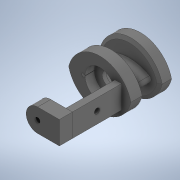
# Autodesk Inventor part: SpoolHolder
Saved by Autodesk Inventor 2022 (Build 260153000, 153)
## iProperties
Created: 2020-03-10
Part Number: SpoolHolder
Material: Generic
Document SubType Name: Modeling
Designer: elmar
Density: 1 g/cm^3
Appearance: Gray
GuideRadius: 25.000 mm
SpoolHolderPlateDiameter: 30.000 mm
CarriageGuideWidth: 10.000 mm
Author: elmar
Autodesk Inventor part; units mm, degrees
ref_plane "YZ Plane" through (0, 0, 0) normal (1, 0, 0) x (0, 1, 0)
ref_plane "XZ Plane" through (0, 0, 0) normal (0, 1, 0) x (-1, 0, 0)
ref_plane "XY Plane" through (0, 0, 0) normal (0, 0, 1) x (1, 0, 0)
sketch "Sketch1" plane through (0, 0, 0) normal (0, 0, 1) x (1, 0, 0)
  circle A0 centre (0, 0) radius 15
  arc A1 (19, 0) -> (-19, 0) centre (0, -4.5333) ccw
  arc A2 (-19, 0) -> (19, 0) centre (0, 4.5333) ccw
  line L0 (-26.6, 0) -> (26.6, 0) projected
  line L1 (0, -21) -> (0, 21) projected
  point P0 (0, 15)
  point P1 (0, -15)
  dimension "SpoolHolderPlateDiameter" = 30
  dimension "d253" = 38
  constraints: 4 point on circle, 3 centre point, 3 point on line, 2 tangent, 1 coincident
  measures "SpoolHolderPlateDiameter" diameter of A0
  measures "d253" distance of A1.end A1.start
extrude "Extrusion1" add sketch "Sketch1" against normal blind 8
sketch "Sketch3" plane through (0, 0, 0) normal (0, 0, -1) x (-1, 0, 0)
  line L0 (-13.2665, 7) -> (-9.2665, 7)
  line L1 (-9.2665, 7) -> (-9.2665, -7)
  line L2 (-9.2665, -7) -> (-13.2665, -7)
  line L3 (-13.2665, -7) -> (-13.2665, 7)
  line L4 (26.6, 0) -> (-26.6, 0) projected
  arc A0 (19, 0) -> (-19, 0) centre (0, -4.5333) ccw projected
  circle A1 centre (0, 0) radius 15
  point P0 (-13.2665, 0)
  dimension "SupportThickness" = 4
  dimension "d254" = 14
  constraints: 8 end point, 2 parallel, 1 coincident, 1 horizontal, 1 midpoint, 1 perpendicular, 1 point on line, 4 other
  measures "SupportThickness" distance of L0.start L0.end
  measures "d254" distance of L0.end L1.end
extrude "Extrusion2" add sketch "Sketch3" against normal blind 30 contours L0 L1 L4 L3 | L4 L1 L2 L3
sketch "Sketch4" plane through (13.2665, 0, -8) normal (1, 0, 0) x (0, 0, 1)
  line L0 (38, 7) -> (38, -7) projected
  line L1 (38, 0) -> (23, 0)
  point P0 (8, 0)
  dimension "HoleHeight" = 15
  constraints: 2 end point, 1 horizontal, 1 midpoint
  measures "HoleHeight" distance of L1.start L1.end
hole "Hole2" at (13.2665, 0, 15) direction (-1, 0, 0) diameter 3.2 depth 4 tip angle 118 clearance for "Flat Head Machine Screw" size "M3" standard "Ansi Metric M Profile"
sketch "Sketch5" plane through (-9.2769, -6.9803, 30) normal (0, 0, 1) x (-1, 0, 0)
  line L0 (-22.5434, -13.9803) -> (-18.5434, -13.9803) projected
  line L1 (-22.5434, 0.0197) -> (-22.5434, -13.9803) projected
  line L2 (-18.5434, 0.0197) -> (-22.5434, 0.0197) projected
  line L3 (-18.5434, -13.9803) -> (-18.5434, 0.0197) projected
  line L4 (-22.5434, -13.9803) -> (-18.5434, -13.9803) projected
  line L5 (-22.5434, -13.9803) -> (2.4566, -13.9803)
  line L6 (2.4566, -13.9803) -> (2.4566, 0.0197)
  line L7 (2.4566, 0.0197) -> (-22.5434, 0.0197)
  line L8 (-22.5434, 0.0197) -> (-22.5434, -13.9803)
  dimension "d255" = 25
  constraints: 8 end point, 2 parallel, 1 collinear, 1 horizontal, 1 perpendicular
  measures "d255" distance of L0.start L5.end
extrude "Extrusion3" add sketch "Sketch5" along normal blind 8
sketch "Sketch6" plane through (-9.2769, -6.9803, 38) normal (0, 0, 1) x (-1, 0, 0)
  circle A0 centre (-9.2769, -6.9803) radius 1.5
  dimension "CableGuideHoleDiameter" = 3
  constraints: 1 centre point, 1 coincident
  measures "CableGuideHoleDiameter" diameter of A0
extrude "Extrusion4" cut sketch "Sketch6" against normal up to surface (8 mm away) draft 30
ref_plane "Work Plane1" through (-13.2769, -6.9803, 38) normal (0, 0, -1) x (1, 0, 0)
ref_plane "Work Plane8" through (-9.2769, -6.9803, 37) normal (0, 0, 1) x (1, 0, 0)
sketch "Sketch10" plane through (-9.2769, -6.9803, 30) normal (0, 0, 1) x (-1, 0, 0)
  line L0 (-22.5434, -6.9803) -> (-18.5434, -6.9803)
  line L1 (-20.5434, -2.6902) -> (-20.5434, -11.2705)
  line L2 (-22.5434, 0.0197) -> (-22.5434, -13.9803) projected
  line L3 (-18.5434, -13.9803) -> (-18.5434, 0.0197) projected
  point P0 (-20.5434, -6.9803)
  point P1 (-22.5434, -6.9803)
  dimension "PinHoleSpacing" = 8.5803
  constraints: 6 midpoint, 4 end point, 1 vertical
  measures "PinHoleSpacing" distance of L1.start L1.end
sketch "Sketch15" plane through (0, 0, -8) normal (0, 0, 1) x (1, 0, 0)
  circle A0 centre (0, 0) radius 5
  line L0 (-26.6, 0) -> (26.6, 0) projected
  arc A1 (15, 0) -> (-15, 0) centre (0, -20) ccw
  arc A2 (-15, 0) -> (15, 0) centre (0, 20) ccw
  circle A3 centre (0, 0) radius 1.5 projected
  circle A4 centre (0, 0) radius 15
  arc A5 (19, 0) -> (-19, 0) centre (0, -4.5333) ccw projected
  dimension "CarriageGuideWidth" = 10
  dimension "GuideRadius" = 25
  constraints: 6 point on circle, 4 centre point, 3 coincident, 2 point on line, 2 tangent, 1 equal radius
  measures "CarriageGuideWidth" diameter of A0
  measures "GuideRadius" radius of A2
extrude "Extrusion5" add sketch "Sketch15" against normal blind 10 contours L0 A3 A0 | L0 A2 A0 | A0 L0 A3 | A0 A1 L0 | A0 L0 A1 | A2 L0 A0 | A3 L0 | L0 A3
split body "Split7" result two bodies by plane through (0, 0, 0) normal (0, 0, 1) first body at (12.7665, 0, 30.8667)
sketch "Sketch26" plane through (-9.2769, -6.9803, 38) normal (0, 0, 1) x (1, 0, 0)
  circle A0 centre (9.2769, 6.9803) radius 6.1188 projected
  circle A1 centre (9.2769, 6.9803) radius 7
  line L0 (-2.4566, -0.0197) -> (22.5434, -0.0197) projected
  line L1 (-2.4566, 13.9803) -> (-2.4566, -0.0197) projected
  line L2 (22.5434, 13.9803) -> (-2.4566, 13.9803) projected
  point P0 (9.2769, -0.0197)
  point P1 (9.2769, 13.9803)
  constraints: 1 centre point, 1 coincident, 1 tangent
extrude "Extrusion9" cut sketch "Sketch26" against normal through all contours A1 L0 L1 L2 bodies 2
chamfer "Chamfer1" distance 2 angle 30 2 edges at (0, -15, -8) (0, 15, -8) measured on face at (0, 14.5, -8) measured on face at (0, -14.5, -8)
ref_plane "Work Plane10" through (0, 0, -7) normal (0, 0, -1) x (-1, 0, 0)
hole "Hole8" at (11.2665, 4.2902, 30) at (11.2665, -4.2902, 30) direction (0, 0, -1) diameter 2.2 depth 37 bodies 2 3
fillet "Fillet2" radius 2 2 edges at (-15, 0, -13) (15, 0, -13)
ref_plane "Work Plane11" through (-7, 0, 30) normal (0, 0, -1) x (-1, 0, 0)
split body "Split8" result two bodies by plane through (-7, 0, 30) normal (0, 0, -1) bodies 2 first body at (9.7665, 0, 4.4667)
ref_plane "Work Plane12" through (16.9371, 0, -8) normal (0, 0, -1) x (-1, 0, 0)
split body "Split9" result two bodies by plane through (16.9371, 0, -8) normal (0, 0, -1) bodies 3 first body at (-0.8434, -4.4855, -11.3333)
sketch "Sketch42" plane through (0, 0, -18) normal (0, 0, -1) x (-1, 0, 0)
  arc A0 (19, 0) -> (-19, 0) centre (0, -4.5333) ccw projected
  arc A1 (-19, 0) -> (19, 0) centre (0, 4.5333) ccw projected
  point P0 (0, 0)
extrude "Extrusion14" add sketch "Sketch42" along normal blind 8 bodies 6
chamfer "Chamfer2" distance 2 angle 30 2 edges at (0, -15, -18) (0, 15, -18) measured on face at (0, 14.5, -18) measured on face at (0, -14.5, -18)
chamfer "Chamfer3" distance 2 angle 30 2 edges at (0, 15, -26) (0, -15, -26) measured on face at (0, 14.5, -26) measured on face at (0, -14.5, -26)
ref_plane "Work Plane13" through (0, 0, -18) normal (0, 0, 1) x (1, 0, 0)
split body "Split10" result two bodies by plane through (0, 0, -18) normal (0, 0, 1) bodies 6 first body at (-0.8434, -4.4855, -11.3333)
sketch "Sketch40" plane through (-9.2769, -6.9803, 30) normal (0, 0, -1) x (-1, 0, 0)
  circle A0 centre (-20.5434, 11.2705) radius 1.1 projected
  circle A1 centre (-20.5434, 2.6902) radius 1.1 projected
  point P0 (-9.2769, 6.9803)
hole "Hole10" at (11.2665, 4.2902, 30) at (11.2665, -4.2902, 30) direction (0, 0, 1) diameter 2 depth 6 tip angle 118 bodies 5
sketch "Sketch35" plane through (0, -20, -26) normal (0, 0, -1) x (-1, 0, 0)
  line L0 (-10, 20) -> (10, 20)
  circle A0 centre (-10, 20) radius 1.5
  circle A1 centre (10, 20) radius 1.5
  point P0 (0, 20)
  point P1 (0, 20)
  dimension "d267" = 20
  dimension "d275" = 3
  constraints: 3 coincident, 2 centre point, 2 end point, 1 equal radius, 1 horizontal, 1 midpoint
  measures "d267" distance of L0.start L0.end
  measures "d275" diameter of A0
hole "Hole12" at (10, 0, -26) at (-10, 0, -26) direction (0, 0, 1) diameter 2 end through all bodies 9 8 7
sketch "Sketch16" plane through (0, 0, 0) normal (0, 0, -1) x (1, 0, 0)
  point P0 (0, 0)
hole "Hole6" at (0, 0, 0) direction (0, 0, -1) diameter 8.4 end through all counterbore diameter 18.01 counterbore depth 5.68 bodies 4 5 7 8 9 clearance for "Hex Head Bolt" size "M8" standard "Ansi Metric M Profile"
equation "\"PinHoleSpacing\" = 0.5 * SupportWidth + 0.5 * SpoolShaftHoleDiameter"
equation "\"d37\" = 55deg"
equation "\"Sketch7_Pitch\" = 1.25"
equation "\"d72\" = 55deg"
equation "\"Sketch11_Pitch\" = 1.25"
equation "\"d111\" = 55deg"
equation "\"Sketch17_Pitch\" = 1.25"
equation "\"d154\" = 55deg"
equation "\"Sketch21_Pitch\" = 1.25"
equation "\"d176\" = 55deg"
equation "\"Sketch23_Pitch\" = 1.25"
equation "\"d200\" = 55deg"
equation "\"Sketch27_Pitch\" = 1.25"
equation "\"d223\" = 55deg"
equation "\"Sketch31_Pitch\" = 1.25"
equation "\"d241\" = 55deg"
equation "\"Sketch33_Pitch\" = 1.25"
equation "\"d285\" = 55deg"
equation "\"Sketch36_Pitch\" = 1.25"
equation "\"d304\" = 55deg"
equation "\"Sketch38_Pitch\" = 1.25"
equation "\"SupportWidth\" = 13.960667"
equation "\"SpoolShaftHoleDiameter\" = 3.2"
